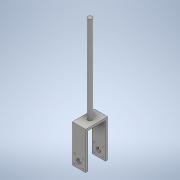
# Autodesk Inventor part: Big Wheel Mount
Saved by Autodesk Inventor 2022 (Build 260153000, 153)
## iProperties
Created: 2021-12-05
Part Number: Big Wheel Mount
Material: Generic
Document SubType Name: Modeling
Designer: Vedic
Density: 1 g/cm^3
Appearance: Default
Author: Vedic
Autodesk Inventor part; units mm, degrees
ref_plane "YZ Plane" through (0, 0, 0) normal (1, 0, 0) x (0, 1, 0)
ref_plane "XZ Plane" through (0, 0, 0) normal (0, 1, 0) x (-1, 0, 0)
ref_plane "XY Plane" through (0, 0, 0) normal (0, 0, 1) x (1, 0, 0)
sketch "Sketch1" plane through (0, 0, 0) normal (0, 1, 0) x (-1, 0, 0)
  line L0 (18.2162, 77.2548) -> (-57.9838, 77.2548)
  line L1 (-57.9838, 77.2548) -> (-57.9838, -24.3452)
  line L2 (-57.9838, -24.3452) -> (18.2162, -24.3452)
  line L3 (18.2162, -24.3452) -> (18.2162, 77.2548)
  point P0 (0, 0)
  dimension "d0" = 101.6
  dimension "d1" = 76.2
  constraints: 8 end point, 2 parallel, 1 horizontal, 1 perpendicular
  measures "d0" distance of L2.end L0.start
  measures "d1" distance of L1.end L2.end
extrude "Extrusion1" add sketch "Sketch1" along normal blind 12.7
sketch "Sketch2" plane through (57.9838, 0, -24.3452) normal (0, 0, -1) x (-1, 0, 0)
  line L0 (0, 0) -> (0, -203.2)
  line L1 (0, -203.2) -> (76.2, -203.2)
  line L2 (0, 0) -> (76.2, 0) projected
  line L3 (76.2, -203.2) -> (76.2, 0)
  line L4 (0, 12.7) -> (76.2, 12.7) projected
  line L5 (0, 0) -> (0, 12.7)
  line L6 (0, 12.7) -> (76.2, 12.7)
  line L7 (76.2, 12.7) -> (76.2, 0)
  point P0 (57.9838, 0)
  dimension "d4" = 90
  dimension "d5" = 203.2
  constraints: 12 end point, 2 equal length, 2 perpendicular, 1 horizontal
  measures "d4" angle of L2 L0
  measures "d5" distance between parallel lines of L2 L1
extrude "Extrusion2" add sketch "Sketch2" along normal blind 12.7
sketch "Sketch3" plane through (-18.2162, 0, 77.2548) normal (0, 0, 1) x (1, 0, 0)
  line L0 (0, 0) -> (0, 12.7) projected
  line L1 (0, 0) -> (0, 12.7)
  line L2 (76.2, 0) -> (76.2, 12.7) projected
  line L3 (0, 12.7) -> (76.2, 12.7)
  line L4 (76.2, 12.7) -> (76.2, 0)
  line L5 (76.2, 0) -> (76.2, -203.2) projected
  line L6 (76.2, 0) -> (76.2, -203.2)
  line L7 (76.2, -203.2) -> (0, -203.2) projected
  line L8 (76.2, -203.2) -> (0, -203.2)
  line L9 (0, -203.2) -> (0, 0)
  point P0 (18.2162, 0)
  constraints: 12 end point, 4 equal length, 2 perpendicular
extrude "Extrusion3" add sketch "Sketch3" along normal blind 12.7
sketch "Sketch4" plane through (0, 12.7, 0) normal (0, 1, 0) x (1, 0, 0)
  line L0 (-18.2162, -77.2548) -> (57.9838, -77.2548) construction
  line L1 (-18.2162, 24.3452) -> (-18.2162, -77.2548) construction
  line L2 (57.9838, -77.2548) -> (-18.2162, -77.2548) construction
  line L3 (-18.2162, -77.2548) -> (-18.2162, 24.3452) construction
  line L4 (-18.2162, 24.3452) -> (57.9838, 24.3452) construction
  line L5 (57.9838, 24.3452) -> (57.9838, -77.2548) construction
  line L6 (57.9838, 24.3452) -> (-18.2162, 24.3452) construction
  line L7 (-18.2162, -26.4548) -> (19.8838, -26.4548) construction
  line L8 (19.8838, -26.4548) -> (19.8838, 24.3452) construction
  line L9 (19.8838, 24.3452) -> (-18.2162, 24.3452) construction
  line L10 (-18.2162, 24.3452) -> (-18.2162, -26.4548) construction
  circle A0 centre (19.8838, -26.4548) radius 12.7
  dimension "d27" = 25.4
  constraints: 16 end point, 4 parallel, 2 horizontal, 2 midpoint, 2 perpendicular, 1 centre point, 1 coincident
  measures "d27" diameter of A0
extrude "Extrusion4" add sketch "Sketch4" along normal blind 508
sketch "Sketch6" plane through (-18.2162, 0, 89.9548) normal (0, 0, 1) x (1, 0, 0)
  line L0 (0, -203.2) -> (76.2, -203.2) construction
  line L1 (38.1, -203.2) -> (76.2, -203.2) construction
  line L2 (76.2, -203.2) -> (76.2, -165.1) construction
  line L3 (76.2, -165.1) -> (38.1, -165.1) construction
  line L4 (38.1, -165.1) -> (38.1, -203.2) construction
  circle A0 centre (38.1, -165.1) radius 12.7
  point P0 (18.2162, 0)
  dimension "d28" = 25.4
  constraints: 8 end point, 2 parallel, 2 perpendicular, 1 centre point, 1 coincident, 1 horizontal, 1 midpoint
  measures "d28" diameter of A0
extrude "Extrusion6" cut sketch "Sketch6" against normal through all
sketch "Sketch7" plane through (-18.2162, 0, 89.9548) normal (0, 0, 1) x (1, 0, 0)
  circle A0 centre (38.1, -165.1) radius 12.7 construction
  circle A1 centre (38.1, -165.1) radius 157.48 construction
  line L0 (38.1, -322.58) -> (38.1, -203.2) construction
  line L1 (0, -203.2) -> (76.2, -203.2) construction
  line L2 (0, 0) -> (0, -203.2) construction
  line L3 (0, -203.2) -> (38.1, -165.1) construction
  line L4 (76.2, -203.2) -> (76.2, 0) construction
  line L5 (38.1, -165.1) -> (76.2, -203.2) construction
  line L6 (38.1, -165.1) -> (0, -127) construction
  line L7 (38.1, -165.1) -> (76.2, -127) construction
  line L8 (12.7, -139.7) -> (63.5, -139.7) construction
  line L9 (63.5, -139.7) -> (63.5, -190.5) construction
  line L10 (63.5, -190.5) -> (12.7, -190.5) construction
  line L11 (12.7, -190.5) -> (12.7, -139.7) construction
  circle A2 centre (12.7, -139.7) radius 3.175
  circle A3 centre (63.5, -139.7) radius 3.175
  circle A4 centre (63.5, -190.5) radius 3.175
  circle A5 centre (12.7, -190.5) radius 3.175
  point P0 (18.2162, 0)
  dimension "d31" = 314.96
  dimension "d32" = 119.38
  dimension "d33" = 50.8
  dimension "d34" = 6.35
  constraints: 18 end point, 6 point on line, 4 centre point, 4 coincident, 4 perpendicular, 3 equal radius, 2 parallel, 1 horizontal, 1 midpoint, 1 vertical alignment, 2 other
  measures "d32" distance of L0.start L0.end
  measures "d33" distance of L9.end L10.end
  measures "d34" diameter of A2
extrude "Extrusion7" cut sketch "Sketch7" against normal through all
body "Solid1"
